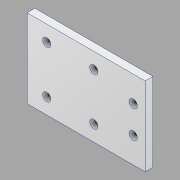
# Autodesk Inventor part: Floor
Saved by Autodesk Inventor 2020 (Build 240168000, 168)
## iProperties
Created: 2019-11-25
Part Number: Floor
Material: Aluminio 6061
Document SubType Name: Modeling
Designer: Gerardo Naranjo
Engineer: Gerardo Naranjo
Density: 2.7 g/cm^3
Appearance: Aluminio - Plano
Title: Floor
Author: Gerardo Naranjo
Autodesk Inventor part; units mm, degrees
ref_plane "YZ Plane" through (0, 0, 0) normal (1, 0, 0) x (0, 1, 0)
ref_plane "XZ Plane" through (0, 0, 0) normal (0, 1, 0) x (-1, 0, 0)
ref_plane "XY Plane" through (0, 0, 0) normal (0, 0, 1) x (1, 0, 0)
sketch "Boceto1" plane through (0, 0, 0) normal (0, 0, 1) x (1, 0, 0)
  line L0 (0, 0) -> (-95.25, 0)
  line L1 (-95.25, 0) -> (-95.25, 63.5)
  line L2 (-95.25, 63.5) -> (0, 63.5)
  line L3 (0, 63.5) -> (0, 0)
  dimension "d0" = 95.25
  dimension "d1" = 63.5
  constraints: 8 end point, 2 parallel, 1 horizontal, 1 perpendicular
  measures "d0" distance of L1.end L2.end
  measures "d1" distance of L0.end L1.end
extrude "Extrusión1" add sketch "Boceto1" along normal blind 6.35
sketch "Boceto2" plane through (0, 0, 6.35) normal (0, 0, 1) x (1, 0, 0)
  line L0 (0, 0) -> (0, 63.5) projected
  line L1 (-111.4017, 31.75) -> (56.4178, 31.75) construction
  line L2 (-95.25, 0) -> (0, 0) projected
  line L3 (0, 63.5) -> (-95.25, 63.5) projected
  point P0 (-79.375, 50.8)
  point P1 (-41.275, 50.8)
  point P2 (-9.525, 42.8625)
  point P3 (-9.525, 20.6375)
  point P4 (-41.275, 12.7)
  point P5 (-79.375, 12.7)
  dimension "d4" = 9.525
  dimension "d5" = 31.75
  dimension "d6" = 38.1
  dimension "d7" = 9.525
  dimension "d8" = 31.75
  dimension "d9" = 38.1
  dimension "d10" = 63.5
  dimension "d11" = 31.75
  dimension "d12" = 22.225
  dimension "d13" = 11.1125
  dimension "d14" = 38.1
  dimension "d15" = 38.1
  dimension "d16" = 19.05
  dimension "d17" = 19.05
  constraints: 2 end point, 1 horizontal
  measures "d4" distance from line of L0 point (-9.525, 42.862)
  measures "d5" horizontal distance of point (-41.275, 50.8) point (-9.525, 42.862)
  measures "d6" distance of point (-79.375, 50.8) point (-41.275, 50.8)
  measures "d7" distance from line of L0 point (-9.525, 20.637)
  measures "d8" horizontal distance of point (-41.275, 12.7) point (-9.525, 20.637)
  measures "d9" distance of point (-79.375, 12.7) point (-41.275, 12.7)
  measures "d10" distance between parallel lines of L2 L3
  measures "d11" distance between parallel lines of L1 L3
  measures "d12" distance of point (-9.525, 20.637) point (-9.525, 42.862)
  measures "d13" distance from line of L1 point (-9.525, 42.862)
  measures "d14" distance of point (-41.275, 12.7) point (-41.275, 50.8)
  measures "d15" distance of point (-79.375, 50.8) point (-79.375, 12.7)
  measures "d16" distance from line of L1 point (-41.275, 50.8)
  measures "d17" distance from line of L1 point (-79.375, 50.8)
hole "Agujero1" at (-79.375, 50.8, 6.35) at (-41.275, 50.8, 6.35) at (-9.525, 42.8625, 6.35) at (-9.525, 20.6375, 6.35) at (-41.275, 12.7, 6.35) at (-79.375, 12.7, 6.35) direction (0, 0, -1) diameter 2.4867 end through all countersink diameter 6.604 countersink angle 82 thread size "5-40 UNC" class "2B" standard "ANSI Unified Screw Threads"
equation "\"d7\" = d4"
equation "\"d8\" = d5"
equation "\"d9\" = d6"
equation "\"d11\" = 0.5 * d10"
equation "\"d13\" = 0.5 * d12"
equation "\"d15\" = d14"
equation "\"d16\" = 0.5 * d14"
equation "\"d17\" = 0.5 * d15"
